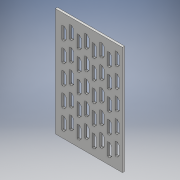
# Autodesk Inventor part: laminarFlowVOLUME50x31cm
Saved by Autodesk Inventor 2017 (Build 210142000, 142)
## iProperties
Created: 2018-08-04
Part Number: laminarFlowVOLUME50x31cm
Material: Generic
Document SubType Name: Modeling
Designer: qwertyuiop1
Density: 1 g/cm^3
Appearance: Default
Author: qwertyuiop1
Autodesk Inventor part; units mm, degrees
ref_plane "YZ Plane" through (0, 0, 0) normal (1, 0, 0) x (0, 1, 0)
ref_plane "XZ Plane" through (0, 0, 0) normal (0, 1, 0) x (-1, 0, 0)
ref_plane "XY Plane" through (0, 0, 0) normal (0, 0, 1) x (1, 0, 0)
sketch "Sketch1" plane through (0, 0, 0) normal (0, 1, 0) x (-1, 0, 0)
  line L0 (-32, 30) -> (-39.1716, 30)
  line L1 (-50, 40.8284) -> (-50, 79.1716)
  line L2 (-39.1716, 90) -> (-32, 90)
  line L3 (-30, 88) -> (-30, 32)
  line L4 (-49.4142, 80.5858) -> (-40.5858, 89.4142)
  line L5 (-40.5858, 30.5858) -> (-49.4142, 39.4142)
  arc A0 (-30, 88) -> (-32, 90) centre (-32, 88) ccw
  arc A1 (-39.1716, 90) -> (-40.5858, 89.4142) centre (-39.1716, 88) ccw
  arc A2 (-49.4142, 80.5858) -> (-50, 79.1716) centre (-48, 79.1716) ccw
  arc A3 (-50, 40.8284) -> (-49.4142, 39.4142) centre (-48, 40.8284) ccw
  arc A4 (-40.5858, 30.5858) -> (-39.1716, 30) centre (-39.1716, 32) ccw
  arc A5 (-32, 30) -> (-30, 32) centre (-32, 32) ccw
  line L6 (-32, 120) -> (-39.1716, 120)
  line L7 (-50, 130.8284) -> (-50, 169.1716)
  line L8 (-39.1716, 180) -> (-32, 180)
  line L9 (-30, 178) -> (-30, 122)
  line L10 (-49.4142, 170.5858) -> (-40.5858, 179.4142)
  line L11 (-40.5858, 120.5858) -> (-49.4142, 129.4142)
  arc A6 (-30, 178) -> (-32, 180) centre (-32, 178) ccw
  arc A7 (-39.1716, 180) -> (-40.5858, 179.4142) centre (-39.1716, 178) ccw
  arc A8 (-49.4142, 170.5858) -> (-50, 169.1716) centre (-48, 169.1716) ccw
  arc A9 (-50, 130.8284) -> (-49.4142, 129.4142) centre (-48, 130.8284) ccw
  arc A10 (-40.5858, 120.5858) -> (-39.1716, 120) centre (-39.1716, 122) ccw
  arc A11 (-32, 120) -> (-30, 122) centre (-32, 122) ccw
  line L12 (-32, 210) -> (-39.1716, 210)
  line L13 (-50, 220.8284) -> (-50, 259.1716)
  line L14 (-39.1716, 270) -> (-32, 270)
  line L15 (-30, 268) -> (-30, 212)
  line L16 (-49.4142, 260.5858) -> (-40.5858, 269.4142)
  line L17 (-40.5858, 210.5858) -> (-49.4142, 219.4142)
  arc A12 (-30, 268) -> (-32, 270) centre (-32, 268) ccw
  arc A13 (-39.1716, 270) -> (-40.5858, 269.4142) centre (-39.1716, 268) ccw
  arc A14 (-49.4142, 260.5858) -> (-50, 259.1716) centre (-48, 259.1716) ccw
  arc A15 (-50, 220.8284) -> (-49.4142, 219.4142) centre (-48, 220.8284) ccw
  arc A16 (-40.5858, 210.5858) -> (-39.1716, 210) centre (-39.1716, 212) ccw
  arc A17 (-32, 210) -> (-30, 212) centre (-32, 212) ccw
  line L18 (-32, 300) -> (-39.1716, 300)
  arc A18 (-50, 310.8284) -> (-49.4142, 309.4142) centre (-48, 310.8284) ccw
  arc A19 (-32, 300) -> (-30, 302) centre (-32, 302) ccw
  arc A20 (-40.5858, 300.5858) -> (-39.1716, 300) centre (-39.1716, 302) ccw
  line L19 (-40.5858, 300.5858) -> (-49.4142, 309.4142)
  line L20 (-50, 310.8284) -> (-50, 349.1716)
  line L21 (-30, 358) -> (-30, 302)
  arc A21 (-49.4142, 350.5858) -> (-50, 349.1716) centre (-48, 349.1716) ccw
  line L22 (-49.4142, 350.5858) -> (-40.5858, 359.4142)
  arc A22 (-39.1716, 360) -> (-40.5858, 359.4142) centre (-39.1716, 358) ccw
  line L23 (-39.1716, 360) -> (-32, 360)
  arc A23 (-30, 358) -> (-32, 360) centre (-32, 358) ccw
  line L24 (-32, 390) -> (-39.1716, 390)
  arc A24 (-40.5858, 390.5858) -> (-39.1716, 390) centre (-39.1716, 392) ccw
  arc A25 (-32, 390) -> (-30, 392) centre (-32, 392) ccw
  line L25 (-40.5858, 390.5858) -> (-49.4142, 399.4142)
  arc A26 (-50, 400.8284) -> (-49.4142, 399.4142) centre (-48, 400.8284) ccw
  line L26 (-30, 448) -> (-30, 392)
  line L27 (-50, 400.8284) -> (-50, 439.1716)
  arc A27 (-49.4142, 440.5858) -> (-50, 439.1716) centre (-48, 439.1716) ccw
  arc A28 (-30, 448) -> (-32, 450) centre (-32, 448) ccw
  line L28 (-39.1716, 450) -> (-32, 450)
  line L29 (-49.4142, 440.5858) -> (-40.5858, 449.4142)
  arc A29 (-39.1716, 450) -> (-40.5858, 449.4142) centre (-39.1716, 448) ccw
  line L30 (0, 0) -> (-309.0433, 0)
  line L31 (-309.0433, 0) -> (-309.0433, 500)
  line L32 (-309.0433, 500) -> (0, 500)
  line L33 (0, 500) -> (0, 0)
  line L34 (-67, 50) -> (-74.1716, 50)
  line L35 (-85, 60.8284) -> (-85, 99.1716)
  line L36 (-74.1716, 110) -> (-67, 110)
  line L37 (-65, 108) -> (-65, 52)
  line L38 (-84.4142, 100.5858) -> (-75.5858, 109.4142)
  line L39 (-75.5858, 50.5858) -> (-84.4142, 59.4142)
  arc A30 (-65, 108) -> (-67, 110) centre (-67, 108) ccw
  arc A31 (-74.1716, 110) -> (-75.5858, 109.4142) centre (-74.1716, 108) ccw
  arc A32 (-84.4142, 100.5858) -> (-85, 99.1716) centre (-83, 99.1716) ccw
  arc A33 (-85, 60.8284) -> (-84.4142, 59.4142) centre (-83, 60.8284) ccw
  arc A34 (-75.5858, 50.5858) -> (-74.1716, 50) centre (-74.1716, 52) ccw
  arc A35 (-67, 50) -> (-65, 52) centre (-67, 52) ccw
  line L40 (-67, 140) -> (-74.1716, 140)
  arc A36 (-85, 150.8284) -> (-84.4142, 149.4142) centre (-83, 150.8284) ccw
  arc A37 (-67, 140) -> (-65, 142) centre (-67, 142) ccw
  arc A38 (-75.5858, 140.5858) -> (-74.1716, 140) centre (-74.1716, 142) ccw
  line L41 (-75.5858, 140.5858) -> (-84.4142, 149.4142)
  line L42 (-85, 150.8284) -> (-85, 189.1716)
  line L43 (-65, 198) -> (-65, 142)
  arc A39 (-84.4142, 190.5858) -> (-85, 189.1716) centre (-83, 189.1716) ccw
  line L44 (-84.4142, 190.5858) -> (-75.5858, 199.4142)
  arc A40 (-74.1716, 200) -> (-75.5858, 199.4142) centre (-74.1716, 198) ccw
  line L45 (-74.1716, 200) -> (-67, 200)
  arc A41 (-65, 198) -> (-67, 200) centre (-67, 198) ccw
  line L46 (-67, 230) -> (-74.1716, 230)
  arc A42 (-85, 240.8284) -> (-84.4142, 239.4142) centre (-83, 240.8284) ccw
  arc A43 (-67, 230) -> (-65, 232) centre (-67, 232) ccw
  arc A44 (-75.5858, 230.5858) -> (-74.1716, 230) centre (-74.1716, 232) ccw
  line L47 (-75.5858, 230.5858) -> (-84.4142, 239.4142)
  line L48 (-85, 240.8284) -> (-85, 279.1716)
  line L49 (-65, 288) -> (-65, 232)
  arc A45 (-84.4142, 280.5858) -> (-85, 279.1716) centre (-83, 279.1716) ccw
  line L50 (-84.4142, 280.5858) -> (-75.5858, 289.4142)
  arc A46 (-74.1716, 290) -> (-75.5858, 289.4142) centre (-74.1716, 288) ccw
  line L51 (-74.1716, 290) -> (-67, 290)
  arc A47 (-65, 288) -> (-67, 290) centre (-67, 288) ccw
  line L52 (-67, 320) -> (-74.1716, 320)
  arc A48 (-75.5858, 320.5858) -> (-74.1716, 320) centre (-74.1716, 322) ccw
  arc A49 (-67, 320) -> (-65, 322) centre (-67, 322) ccw
  line L53 (-75.5858, 320.5858) -> (-84.4142, 329.4142)
  arc A50 (-85, 330.8284) -> (-84.4142, 329.4142) centre (-83, 330.8284) ccw
  line L54 (-65, 378) -> (-65, 322)
  line L55 (-85, 330.8284) -> (-85, 369.1716)
  arc A51 (-84.4142, 370.5858) -> (-85, 369.1716) centre (-83, 369.1716) ccw
  arc A52 (-65, 378) -> (-67, 380) centre (-67, 378) ccw
  line L56 (-74.1716, 380) -> (-67, 380)
  line L57 (-84.4142, 370.5858) -> (-75.5858, 379.4142)
  arc A53 (-74.1716, 380) -> (-75.5858, 379.4142) centre (-74.1716, 378) ccw
  line L58 (-67, 410) -> (-74.1716, 410)
  arc A54 (-75.5858, 410.5858) -> (-74.1716, 410) centre (-74.1716, 412) ccw
  arc A55 (-67, 410) -> (-65, 412) centre (-67, 412) ccw
  line L59 (-75.5858, 410.5858) -> (-84.4142, 419.4142)
  line L60 (-65, 468) -> (-65, 412)
  line L61 (-85, 420.8284) -> (-85, 459.1716)
  arc A56 (-85, 420.8284) -> (-84.4142, 419.4142) centre (-83, 420.8284) ccw
  arc A57 (-84.4142, 460.5858) -> (-85, 459.1716) centre (-83, 459.1716) ccw
  line L62 (-84.4142, 460.5858) -> (-75.5858, 469.4142)
  arc A58 (-74.1716, 470) -> (-75.5858, 469.4142) centre (-74.1716, 468) ccw
  line L63 (-74.1716, 470) -> (-67, 470)
  arc A59 (-65, 468) -> (-67, 470) centre (-67, 468) ccw
  line L64 (-102, 30) -> (-109.1716, 30)
  line L65 (-120, 40.8284) -> (-120, 79.1716)
  line L66 (-109.1716, 90) -> (-102, 90)
  line L67 (-100, 88) -> (-100, 32)
  line L68 (-119.4142, 80.5858) -> (-110.5858, 89.4142)
  line L69 (-110.5858, 30.5858) -> (-119.4142, 39.4142)
  arc A60 (-100, 88) -> (-102, 90) centre (-102, 88) ccw
  arc A61 (-109.1716, 90) -> (-110.5858, 89.4142) centre (-109.1716, 88) ccw
  arc A62 (-119.4142, 80.5858) -> (-120, 79.1716) centre (-118, 79.1716) ccw
  arc A63 (-120, 40.8284) -> (-119.4142, 39.4142) centre (-118, 40.8284) ccw
  arc A64 (-110.5858, 30.5858) -> (-109.1716, 30) centre (-109.1716, 32) ccw
  arc A65 (-102, 30) -> (-100, 32) centre (-102, 32) ccw
  line L70 (-102, 120) -> (-109.1716, 120)
  arc A66 (-120, 130.8284) -> (-119.4142, 129.4142) centre (-118, 130.8284) ccw
  arc A67 (-102, 120) -> (-100, 122) centre (-102, 122) ccw
  arc A68 (-110.5858, 120.5858) -> (-109.1716, 120) centre (-109.1716, 122) ccw
  line L71 (-110.5858, 120.5858) -> (-119.4142, 129.4142)
  line L72 (-120, 130.8284) -> (-120, 169.1716)
  line L73 (-100, 178) -> (-100, 122)
  arc A69 (-119.4142, 170.5858) -> (-120, 169.1716) centre (-118, 169.1716) ccw
  line L74 (-119.4142, 170.5858) -> (-110.5858, 179.4142)
  arc A70 (-109.1716, 180) -> (-110.5858, 179.4142) centre (-109.1716, 178) ccw
  line L75 (-109.1716, 180) -> (-102, 180)
  arc A71 (-100, 178) -> (-102, 180) centre (-102, 178) ccw
  line L76 (-102, 210) -> (-109.1716, 210)
  arc A72 (-120, 220.8284) -> (-119.4142, 219.4142) centre (-118, 220.8284) ccw
  arc A73 (-102, 210) -> (-100, 212) centre (-102, 212) ccw
  arc A74 (-110.5858, 210.5858) -> (-109.1716, 210) centre (-109.1716, 212) ccw
  line L77 (-110.5858, 210.5858) -> (-119.4142, 219.4142)
  line L78 (-120, 220.8284) -> (-120, 259.1716)
  line L79 (-100, 268) -> (-100, 212)
  arc A75 (-119.4142, 260.5858) -> (-120, 259.1716) centre (-118, 259.1716) ccw
  line L80 (-119.4142, 260.5858) -> (-110.5858, 269.4142)
  arc A76 (-109.1716, 270) -> (-110.5858, 269.4142) centre (-109.1716, 268) ccw
  line L81 (-109.1716, 270) -> (-102, 270)
  arc A77 (-100, 268) -> (-102, 270) centre (-102, 268) ccw
  line L82 (-102, 300) -> (-109.1716, 300)
  arc A78 (-110.5858, 300.5858) -> (-109.1716, 300) centre (-109.1716, 302) ccw
  arc A79 (-102, 300) -> (-100, 302) centre (-102, 302) ccw
  line L83 (-110.5858, 300.5858) -> (-119.4142, 309.4142)
  arc A80 (-120, 310.8284) -> (-119.4142, 309.4142) centre (-118, 310.8284) ccw
  line L84 (-100, 358) -> (-100, 302)
  line L85 (-120, 310.8284) -> (-120, 349.1716)
  arc A81 (-119.4142, 350.5858) -> (-120, 349.1716) centre (-118, 349.1716) ccw
  arc A82 (-100, 358) -> (-102, 360) centre (-102, 358) ccw
  line L86 (-109.1716, 360) -> (-102, 360)
  line L87 (-119.4142, 350.5858) -> (-110.5858, 359.4142)
  arc A83 (-109.1716, 360) -> (-110.5858, 359.4142) centre (-109.1716, 358) ccw
  line L88 (-102, 390) -> (-109.1716, 390)
  arc A84 (-110.5858, 390.5858) -> (-109.1716, 390) centre (-109.1716, 392) ccw
  arc A85 (-102, 390) -> (-100, 392) centre (-102, 392) ccw
  line L89 (-110.5858, 390.5858) -> (-119.4142, 399.4142)
  line L90 (-100, 448) -> (-100, 392)
  line L91 (-120, 400.8284) -> (-120, 439.1716)
  arc A86 (-120, 400.8284) -> (-119.4142, 399.4142) centre (-118, 400.8284) ccw
  arc A87 (-119.4142, 440.5858) -> (-120, 439.1716) centre (-118, 439.1716) ccw
  line L92 (-119.4142, 440.5858) -> (-110.5858, 449.4142)
  arc A88 (-109.1716, 450) -> (-110.5858, 449.4142) centre (-109.1716, 448) ccw
  line L93 (-109.1716, 450) -> (-102, 450)
  arc A89 (-100, 448) -> (-102, 450) centre (-102, 448) ccw
  arc A90 (-155, 420.8284) -> (-154.4142, 419.4142) centre (-153, 420.8284) ccw
  line L94 (-155, 420.8284) -> (-155, 459.1716)
  line L95 (-135, 468) -> (-135, 412)
  line L96 (-144.1716, 470) -> (-137, 470)
  arc A91 (-145.5858, 410.5858) -> (-144.1716, 410) centre (-144.1716, 412) ccw
  arc A92 (-137, 410) -> (-135, 412) centre (-137, 412) ccw
  line L97 (-145.5858, 410.5858) -> (-154.4142, 419.4142)
  arc A93 (-154.4142, 460.5858) -> (-155, 459.1716) centre (-153, 459.1716) ccw
  line L98 (-154.4142, 460.5858) -> (-145.5858, 469.4142)
  arc A94 (-135, 468) -> (-137, 470) centre (-137, 468) ccw
  arc A95 (-144.1716, 470) -> (-145.5858, 469.4142) centre (-144.1716, 468) ccw
  line L99 (-137, 50) -> (-144.1716, 50)
  arc A96 (-154.4142, 280.5858) -> (-155, 279.1716) centre (-153, 279.1716) ccw
  line L100 (-154.4142, 280.5858) -> (-145.5858, 289.4142)
  arc A97 (-144.1716, 290) -> (-145.5858, 289.4142) centre (-144.1716, 288) ccw
  arc A98 (-154.4142, 370.5858) -> (-155, 369.1716) centre (-153, 369.1716) ccw
  arc A99 (-155, 330.8284) -> (-154.4142, 329.4142) centre (-153, 330.8284) ccw
  arc A100 (-144.1716, 380) -> (-145.5858, 379.4142) centre (-144.1716, 378) ccw
  line L101 (-145.5858, 50.5858) -> (-154.4142, 59.4142)
  line L102 (-155, 60.8284) -> (-155, 99.1716)
  line L103 (-154.4142, 100.5858) -> (-145.5858, 109.4142)
  line L104 (-135, 108) -> (-135, 52)
  line L105 (-144.1716, 110) -> (-137, 110)
  line L106 (-155, 330.8284) -> (-155, 369.1716)
  line L107 (-144.1716, 290) -> (-137, 290)
  line L108 (-137, 320) -> (-144.1716, 320)
  line L109 (-137, 410) -> (-144.1716, 410)
  arc A101 (-137, 320) -> (-135, 322) centre (-137, 322) ccw
  arc A102 (-135, 288) -> (-137, 290) centre (-137, 288) ccw
  line L110 (-154.4142, 370.5858) -> (-145.5858, 379.4142)
  line L111 (-145.5858, 320.5858) -> (-154.4142, 329.4142)
  arc A103 (-135, 378) -> (-137, 380) centre (-137, 378) ccw
  arc A104 (-135, 108) -> (-137, 110) centre (-137, 108) ccw
  arc A105 (-144.1716, 110) -> (-145.5858, 109.4142) centre (-144.1716, 108) ccw
  arc A106 (-154.4142, 100.5858) -> (-155, 99.1716) centre (-153, 99.1716) ccw
  arc A107 (-155, 240.8284) -> (-154.4142, 239.4142) centre (-153, 240.8284) ccw
  arc A108 (-155, 60.8284) -> (-154.4142, 59.4142) centre (-153, 60.8284) ccw
  arc A109 (-145.5858, 50.5858) -> (-144.1716, 50) centre (-144.1716, 52) ccw
  arc A110 (-137, 50) -> (-135, 52) centre (-137, 52) ccw
  line L112 (-135, 378) -> (-135, 322)
  line L113 (-144.1716, 380) -> (-137, 380)
  line L114 (-137, 230) -> (-144.1716, 230)
  line L115 (-155, 240.8284) -> (-155, 279.1716)
  line L116 (-145.5858, 230.5858) -> (-154.4142, 239.4142)
  line L117 (-135, 288) -> (-135, 232)
  line L118 (-155, 150.8284) -> (-155, 189.1716)
  line L119 (-135, 198) -> (-135, 142)
  line L120 (-145.5858, 140.5858) -> (-154.4142, 149.4142)
  arc A111 (-155, 150.8284) -> (-154.4142, 149.4142) centre (-153, 150.8284) ccw
  arc A112 (-137, 140) -> (-135, 142) centre (-137, 142) ccw
  arc A113 (-145.5858, 140.5858) -> (-144.1716, 140) centre (-144.1716, 142) ccw
  line L121 (-137, 140) -> (-144.1716, 140)
  arc A114 (-145.5858, 320.5858) -> (-144.1716, 320) centre (-144.1716, 322) ccw
  arc A115 (-137, 230) -> (-135, 232) centre (-137, 232) ccw
  arc A116 (-145.5858, 230.5858) -> (-144.1716, 230) centre (-144.1716, 232) ccw
  line L122 (-144.1716, 200) -> (-137, 200)
  arc A117 (-144.1716, 200) -> (-145.5858, 199.4142) centre (-144.1716, 198) ccw
  arc A118 (-135, 198) -> (-137, 200) centre (-137, 198) ccw
  line L123 (-154.4142, 190.5858) -> (-145.5858, 199.4142)
  arc A119 (-154.4142, 190.5858) -> (-155, 189.1716) centre (-153, 189.1716) ccw
  line L124 (-172, 30) -> (-179.1716, 30)
  line L125 (-190, 40.8284) -> (-190, 79.1716)
  line L126 (-179.1716, 90) -> (-172, 90)
  line L127 (-170, 88) -> (-170, 32)
  line L128 (-189.4142, 80.5858) -> (-180.5858, 89.4142)
  line L129 (-180.5858, 30.5858) -> (-189.4142, 39.4142)
  arc A120 (-170, 88) -> (-172, 90) centre (-172, 88) ccw
  arc A121 (-179.1716, 90) -> (-180.5858, 89.4142) centre (-179.1716, 88) ccw
  arc A122 (-189.4142, 80.5858) -> (-190, 79.1716) centre (-188, 79.1716) ccw
  arc A123 (-190, 40.8284) -> (-189.4142, 39.4142) centre (-188, 40.8284) ccw
  arc A124 (-180.5858, 30.5858) -> (-179.1716, 30) centre (-179.1716, 32) ccw
  arc A125 (-172, 30) -> (-170, 32) centre (-172, 32) ccw
  line L130 (-172, 120) -> (-179.1716, 120)
  arc A126 (-190, 130.8284) -> (-189.4142, 129.4142) centre (-188, 130.8284) ccw
  arc A127 (-172, 120) -> (-170, 122) centre (-172, 122) ccw
  arc A128 (-180.5858, 120.5858) -> (-179.1716, 120) centre (-179.1716, 122) ccw
  line L131 (-180.5858, 120.5858) -> (-189.4142, 129.4142)
  line L132 (-190, 130.8284) -> (-190, 169.1716)
  line L133 (-170, 178) -> (-170, 122)
  arc A129 (-189.4142, 170.5858) -> (-190, 169.1716) centre (-188, 169.1716) ccw
  line L134 (-189.4142, 170.5858) -> (-180.5858, 179.4142)
  arc A130 (-179.1716, 180) -> (-180.5858, 179.4142) centre (-179.1716, 178) ccw
  line L135 (-179.1716, 180) -> (-172, 180)
  arc A131 (-170, 178) -> (-172, 180) centre (-172, 178) ccw
  line L136 (-172, 210) -> (-179.1716, 210)
  arc A132 (-190, 220.8284) -> (-189.4142, 219.4142) centre (-188, 220.8284) ccw
  arc A133 (-172, 210) -> (-170, 212) centre (-172, 212) ccw
  arc A134 (-180.5858, 210.5858) -> (-179.1716, 210) centre (-179.1716, 212) ccw
  line L137 (-180.5858, 210.5858) -> (-189.4142, 219.4142)
  line L138 (-190, 220.8284) -> (-190, 259.1716)
  line L139 (-170, 268) -> (-170, 212)
  arc A135 (-189.4142, 260.5858) -> (-190, 259.1716) centre (-188, 259.1716) ccw
  line L140 (-189.4142, 260.5858) -> (-180.5858, 269.4142)
  arc A136 (-179.1716, 270) -> (-180.5858, 269.4142) centre (-179.1716, 268) ccw
  line L141 (-179.1716, 270) -> (-172, 270)
  arc A137 (-170, 268) -> (-172, 270) centre (-172, 268) ccw
  line L142 (-172, 300) -> (-179.1716, 300)
  arc A138 (-180.5858, 300.5858) -> (-179.1716, 300) centre (-179.1716, 302) ccw
  arc A139 (-172, 300) -> (-170, 302) centre (-172, 302) ccw
  line L143 (-180.5858, 300.5858) -> (-189.4142, 309.4142)
  arc A140 (-190, 310.8284) -> (-189.4142, 309.4142) centre (-188, 310.8284) ccw
  line L144 (-170, 358) -> (-170, 302)
  line L145 (-190, 310.8284) -> (-190, 349.1716)
  arc A141 (-189.4142, 350.5858) -> (-190, 349.1716) centre (-188, 349.1716) ccw
  arc A142 (-170, 358) -> (-172, 360) centre (-172, 358) ccw
  line L146 (-179.1716, 360) -> (-172, 360)
  line L147 (-189.4142, 350.5858) -> (-180.5858, 359.4142)
  arc A143 (-179.1716, 360) -> (-180.5858, 359.4142) centre (-179.1716, 358) ccw
  line L148 (-172, 390) -> (-179.1716, 390)
  arc A144 (-180.5858, 390.5858) -> (-179.1716, 390) centre (-179.1716, 392) ccw
  arc A145 (-172, 390) -> (-170, 392) centre (-172, 392) ccw
  line L149 (-180.5858, 390.5858) -> (-189.4142, 399.4142)
  line L150 (-170, 448) -> (-170, 392)
  line L151 (-190, 400.8284) -> (-190, 439.1716)
  arc A146 (-190, 400.8284) -> (-189.4142, 399.4142) centre (-188, 400.8284) ccw
  arc A147 (-189.4142, 440.5858) -> (-190, 439.1716) centre (-188, 439.1716) ccw
  line L152 (-189.4142, 440.5858) -> (-180.5858, 449.4142)
  arc A148 (-179.1716, 450) -> (-180.5858, 449.4142) centre (-179.1716, 448) ccw
  line L153 (-179.1716, 450) -> (-172, 450)
  arc A149 (-170, 448) -> (-172, 450) centre (-172, 448) ccw
  arc A150 (-225, 420.8284) -> (-224.4142, 419.4142) centre (-223, 420.8284) ccw
  line L154 (-225, 420.8284) -> (-225, 459.1716)
  line L155 (-205, 468) -> (-205, 412)
  line L156 (-214.1716, 470) -> (-207, 470)
  arc A151 (-215.5858, 410.5858) -> (-214.1716, 410) centre (-214.1716, 412) ccw
  arc A152 (-207, 410) -> (-205, 412) centre (-207, 412) ccw
  line L157 (-215.5858, 410.5858) -> (-224.4142, 419.4142)
  arc A153 (-224.4142, 460.5858) -> (-225, 459.1716) centre (-223, 459.1716) ccw
  line L158 (-224.4142, 460.5858) -> (-215.5858, 469.4142)
  arc A154 (-205, 468) -> (-207, 470) centre (-207, 468) ccw
  arc A155 (-214.1716, 470) -> (-215.5858, 469.4142) centre (-214.1716, 468) ccw
  line L159 (-207, 50) -> (-214.1716, 50)
  arc A156 (-224.4142, 280.5858) -> (-225, 279.1716) centre (-223, 279.1716) ccw
  line L160 (-224.4142, 280.5858) -> (-215.5858, 289.4142)
  arc A157 (-214.1716, 290) -> (-215.5858, 289.4142) centre (-214.1716, 288) ccw
  arc A158 (-224.4142, 370.5858) -> (-225, 369.1716) centre (-223, 369.1716) ccw
  arc A159 (-225, 330.8284) -> (-224.4142, 329.4142) centre (-223, 330.8284) ccw
  arc A160 (-214.1716, 380) -> (-215.5858, 379.4142) centre (-214.1716, 378) ccw
  line L161 (-215.5858, 50.5858) -> (-224.4142, 59.4142)
  line L162 (-225, 60.8284) -> (-225, 99.1716)
  line L163 (-224.4142, 100.5858) -> (-215.5858, 109.4142)
  line L164 (-205, 108) -> (-205, 52)
  line L165 (-214.1716, 110) -> (-207, 110)
  line L166 (-225, 330.8284) -> (-225, 369.1716)
  line L167 (-214.1716, 290) -> (-207, 290)
  line L168 (-207, 320) -> (-214.1716, 320)
  line L169 (-207, 410) -> (-214.1716, 410)
  arc A161 (-207, 320) -> (-205, 322) centre (-207, 322) ccw
  arc A162 (-205, 288) -> (-207, 290) centre (-207, 288) ccw
  line L170 (-224.4142, 370.5858) -> (-215.5858, 379.4142)
  line L171 (-215.5858, 320.5858) -> (-224.4142, 329.4142)
  arc A163 (-205, 378) -> (-207, 380) centre (-207, 378) ccw
  arc A164 (-205, 108) -> (-207, 110) centre (-207, 108) ccw
  arc A165 (-214.1716, 110) -> (-215.5858, 109.4142) centre (-214.1716, 108) ccw
  arc A166 (-224.4142, 100.5858) -> (-225, 99.1716) centre (-223, 99.1716) ccw
  arc A167 (-225, 240.8284) -> (-224.4142, 239.4142) centre (-223, 240.8284) ccw
  arc A168 (-225, 60.8284) -> (-224.4142, 59.4142) centre (-223, 60.8284) ccw
  arc A169 (-215.5858, 50.5858) -> (-214.1716, 50) centre (-214.1716, 52) ccw
  arc A170 (-207, 50) -> (-205, 52) centre (-207, 52) ccw
  line L172 (-205, 378) -> (-205, 322)
  line L173 (-214.1716, 380) -> (-207, 380)
  line L174 (-207, 230) -> (-214.1716, 230)
  line L175 (-225, 240.8284) -> (-225, 279.1716)
  line L176 (-215.5858, 230.5858) -> (-224.4142, 239.4142)
  line L177 (-205, 288) -> (-205, 232)
  line L178 (-225, 150.8284) -> (-225, 189.1716)
  line L179 (-205, 198) -> (-205, 142)
  line L180 (-215.5858, 140.5858) -> (-224.4142, 149.4142)
  arc A171 (-225, 150.8284) -> (-224.4142, 149.4142) centre (-223, 150.8284) ccw
  arc A172 (-207, 140) -> (-205, 142) centre (-207, 142) ccw
  arc A173 (-215.5858, 140.5858) -> (-214.1716, 140) centre (-214.1716, 142) ccw
  line L181 (-207, 140) -> (-214.1716, 140)
  arc A174 (-215.5858, 320.5858) -> (-214.1716, 320) centre (-214.1716, 322) ccw
  arc A175 (-207, 230) -> (-205, 232) centre (-207, 232) ccw
  arc A176 (-215.5858, 230.5858) -> (-214.1716, 230) centre (-214.1716, 232) ccw
  line L182 (-214.1716, 200) -> (-207, 200)
  arc A177 (-214.1716, 200) -> (-215.5858, 199.4142) centre (-214.1716, 198) ccw
  arc A178 (-205, 198) -> (-207, 200) centre (-207, 198) ccw
  line L183 (-224.4142, 190.5858) -> (-215.5858, 199.4142)
  arc A179 (-224.4142, 190.5858) -> (-225, 189.1716) centre (-223, 189.1716) ccw
  line L184 (-242, 30) -> (-249.1716, 30)
  line L185 (-260, 40.8284) -> (-260, 79.1716)
  line L186 (-249.1716, 90) -> (-242, 90)
  line L187 (-240, 88) -> (-240, 32)
  line L188 (-259.4142, 80.5858) -> (-250.5858, 89.4142)
  line L189 (-250.5858, 30.5858) -> (-259.4142, 39.4142)
  arc A180 (-240, 88) -> (-242, 90) centre (-242, 88) ccw
  arc A181 (-249.1716, 90) -> (-250.5858, 89.4142) centre (-249.1716, 88) ccw
  arc A182 (-259.4142, 80.5858) -> (-260, 79.1716) centre (-258, 79.1716) ccw
  arc A183 (-260, 40.8284) -> (-259.4142, 39.4142) centre (-258, 40.8284) ccw
  arc A184 (-250.5858, 30.5858) -> (-249.1716, 30) centre (-249.1716, 32) ccw
  arc A185 (-242, 30) -> (-240, 32) centre (-242, 32) ccw
  line L190 (-242, 120) -> (-249.1716, 120)
  arc A186 (-260, 130.8284) -> (-259.4142, 129.4142) centre (-258, 130.8284) ccw
  arc A187 (-242, 120) -> (-240, 122) centre (-242, 122) ccw
  arc A188 (-250.5858, 120.5858) -> (-249.1716, 120) centre (-249.1716, 122) ccw
  line L191 (-250.5858, 120.5858) -> (-259.4142, 129.4142)
  line L192 (-260, 130.8284) -> (-260, 169.1716)
  line L193 (-240, 178) -> (-240, 122)
  arc A189 (-259.4142, 170.5858) -> (-260, 169.1716) centre (-258, 169.1716) ccw
  line L194 (-259.4142, 170.5858) -> (-250.5858, 179.4142)
  arc A190 (-249.1716, 180) -> (-250.5858, 179.4142) centre (-249.1716, 178) ccw
  line L195 (-249.1716, 180) -> (-242, 180)
  arc A191 (-240, 178) -> (-242, 180) centre (-242, 178) ccw
  line L196 (-242, 210) -> (-249.1716, 210)
  arc A192 (-260, 220.8284) -> (-259.4142, 219.4142) centre (-258, 220.8284) ccw
  arc A193 (-242, 210) -> (-240, 212) centre (-242, 212) ccw
  arc A194 (-250.5858, 210.5858) -> (-249.1716, 210) centre (-249.1716, 212) ccw
  line L197 (-250.5858, 210.5858) -> (-259.4142, 219.4142)
  line L198 (-260, 220.8284) -> (-260, 259.1716)
  line L199 (-240, 268) -> (-240, 212)
  arc A195 (-259.4142, 260.5858) -> (-260, 259.1716) centre (-258, 259.1716) ccw
  line L200 (-259.4142, 260.5858) -> (-250.5858, 269.4142)
  arc A196 (-249.1716, 270) -> (-250.5858, 269.4142) centre (-249.1716, 268) ccw
  line L201 (-249.1716, 270) -> (-242, 270)
  arc A197 (-240, 268) -> (-242, 270) centre (-242, 268) ccw
  line L202 (-242, 300) -> (-249.1716, 300)
  arc A198 (-250.5858, 300.5858) -> (-249.1716, 300) centre (-249.1716, 302) ccw
  arc A199 (-242, 300) -> (-240, 302) centre (-242, 302) ccw
  line L203 (-250.5858, 300.5858) -> (-259.4142, 309.4142)
  arc A200 (-260, 310.8284) -> (-259.4142, 309.4142) centre (-258, 310.8284) ccw
  line L204 (-240, 358) -> (-240, 302)
  line L205 (-260, 310.8284) -> (-260, 349.1716)
  arc A201 (-259.4142, 350.5858) -> (-260, 349.1716) centre (-258, 349.1716) ccw
  arc A202 (-240, 358) -> (-242, 360) centre (-242, 358) ccw
  line L206 (-249.1716, 360) -> (-242, 360)
  line L207 (-259.4142, 350.5858) -> (-250.5858, 359.4142)
  arc A203 (-249.1716, 360) -> (-250.5858, 359.4142) centre (-249.1716, 358) ccw
  line L208 (-242, 390) -> (-249.1716, 390)
  arc A204 (-250.5858, 390.5858) -> (-249.1716, 390) centre (-249.1716, 392) ccw
  arc A205 (-242, 390) -> (-240, 392) centre (-242, 392) ccw
  line L209 (-250.5858, 390.5858) -> (-259.4142, 399.4142)
  line L210 (-240, 448) -> (-240, 392)
  line L211 (-260, 400.8284) -> (-260, 439.1716)
  arc A206 (-260, 400.8284) -> (-259.4142, 399.4142) centre (-258, 400.8284) ccw
  arc A207 (-259.4142, 440.5858) -> (-260, 439.1716) centre (-258, 439.1716) ccw
  line L212 (-259.4142, 440.5858) -> (-250.5858, 449.4142)
  arc A208 (-249.1716, 450) -> (-250.5858, 449.4142) centre (-249.1716, 448) ccw
  line L213 (-249.1716, 450) -> (-242, 450)
  arc A209 (-240, 448) -> (-242, 450) centre (-242, 448) ccw
  arc A210 (-295, 420.8284) -> (-294.4142, 419.4142) centre (-293, 420.8284) ccw
  line L214 (-295, 420.8284) -> (-295, 459.1716)
  line L215 (-275, 468) -> (-275, 412)
  line L216 (-284.1716, 470) -> (-277, 470)
  arc A211 (-285.5858, 410.5858) -> (-284.1716, 410) centre (-284.1716, 412) ccw
  arc A212 (-277, 410) -> (-275, 412) centre (-277, 412) ccw
  line L217 (-285.5858, 410.5858) -> (-294.4142, 419.4142)
  arc A213 (-294.4142, 460.5858) -> (-295, 459.1716) centre (-293, 459.1716) ccw
  line L218 (-294.4142, 460.5858) -> (-285.5858, 469.4142)
  arc A214 (-275, 468) -> (-277, 470) centre (-277, 468) ccw
  arc A215 (-284.1716, 470) -> (-285.5858, 469.4142) centre (-284.1716, 468) ccw
  line L219 (-277, 50) -> (-284.1716, 50)
  arc A216 (-294.4142, 280.5858) -> (-295, 279.1716) centre (-293, 279.1716) ccw
  line L220 (-294.4142, 280.5858) -> (-285.5858, 289.4142)
  arc A217 (-284.1716, 290) -> (-285.5858, 289.4142) centre (-284.1716, 288) ccw
  arc A218 (-294.4142, 370.5858) -> (-295, 369.1716) centre (-293, 369.1716) ccw
  arc A219 (-295, 330.8284) -> (-294.4142, 329.4142) centre (-293, 330.8284) ccw
  arc A220 (-284.1716, 380) -> (-285.5858, 379.4142) centre (-284.1716, 378) ccw
  line L221 (-285.5858, 50.5858) -> (-294.4142, 59.4142)
  line L222 (-295, 60.8284) -> (-295, 99.1716)
  line L223 (-294.4142, 100.5858) -> (-285.5858, 109.4142)
  line L224 (-275, 108) -> (-275, 52)
  line L225 (-284.1716, 110) -> (-277, 110)
  line L226 (-295, 330.8284) -> (-295, 369.1716)
  line L227 (-284.1716, 290) -> (-277, 290)
  line L228 (-277, 320) -> (-284.1716, 320)
  line L229 (-277, 410) -> (-284.1716, 410)
  arc A221 (-277, 320) -> (-275, 322) centre (-277, 322) ccw
  arc A222 (-275, 288) -> (-277, 290) centre (-277, 288) ccw
  line L230 (-294.4142, 370.5858) -> (-285.5858, 379.4142)
  line L231 (-285.5858, 320.5858) -> (-294.4142, 329.4142)
  arc A223 (-275, 378) -> (-277, 380) centre (-277, 378) ccw
  arc A224 (-275, 108) -> (-277, 110) centre (-277, 108) ccw
  arc A225 (-284.1716, 110) -> (-285.5858, 109.4142) centre (-284.1716, 108) ccw
  arc A226 (-294.4142, 100.5858) -> (-295, 99.1716) centre (-293, 99.1716) ccw
  arc A227 (-295, 240.8284) -> (-294.4142, 239.4142) centre (-293, 240.8284) ccw
  arc A228 (-295, 60.8284) -> (-294.4142, 59.4142) centre (-293, 60.8284) ccw
  arc A229 (-285.5858, 50.5858) -> (-284.1716, 50) centre (-284.1716, 52) ccw
  arc A230 (-277, 50) -> (-275, 52) centre (-277, 52) ccw
  line L232 (-275, 378) -> (-275, 322)
  line L233 (-284.1716, 380) -> (-277, 380)
  line L234 (-277, 230) -> (-284.1716, 230)
  line L235 (-295, 240.8284) -> (-295, 279.1716)
  line L236 (-285.5858, 230.5858) -> (-294.4142, 239.4142)
  line L237 (-275, 288) -> (-275, 232)
  line L238 (-295, 150.8284) -> (-295, 189.1716)
  line L239 (-275, 198) -> (-275, 142)
  line L240 (-285.5858, 140.5858) -> (-294.4142, 149.4142)
  arc A231 (-295, 150.8284) -> (-294.4142, 149.4142) centre (-293, 150.8284) ccw
  arc A232 (-277, 140) -> (-275, 142) centre (-277, 142) ccw
  arc A233 (-285.5858, 140.5858) -> (-284.1716, 140) centre (-284.1716, 142) ccw
  line L241 (-277, 140) -> (-284.1716, 140)
  arc A234 (-285.5858, 320.5858) -> (-284.1716, 320) centre (-284.1716, 322) ccw
  arc A235 (-277, 230) -> (-275, 232) centre (-277, 232) ccw
  arc A236 (-285.5858, 230.5858) -> (-284.1716, 230) centre (-284.1716, 232) ccw
  line L242 (-284.1716, 200) -> (-277, 200)
  arc A237 (-284.1716, 200) -> (-285.5858, 199.4142) centre (-284.1716, 198) ccw
  arc A238 (-275, 198) -> (-277, 200) centre (-277, 198) ccw
  line L243 (-294.4142, 190.5858) -> (-285.5858, 199.4142)
  arc A239 (-294.4142, 190.5858) -> (-295, 189.1716) centre (-293, 189.1716) ccw
  point P0 (-50, 90)
  point P1 (-50, 30)
  point P2 (-30, 90)
  point P3 (-50, 80)
  point P4 (-40, 90)
  point P5 (-40, 30)
  point P6 (-50, 40)
  point P7 (-32, 180)
  point P8 (-32, 155.0655)
  point P9 (-32, 392)
  point P10 (-50, 180)
  point P11 (-50, 120)
  point P12 (-30, 180)
  point P13 (-50, 170)
  point P14 (-40, 180)
  point P15 (-40, 120)
  point P16 (-50, 130)
  point P17 (-50, 270)
  point P18 (-50, 210)
  point P19 (-30, 270)
  point P20 (-50, 260)
  point P21 (-40, 270)
  point P22 (-40, 210)
  point P23 (-50, 220)
  point P24 (-50, 300)
  point P25 (-50, 310)
  point P26 (-40, 300)
  point P27 (-50, 360)
  point P28 (-30, 360)
  point P29 (-50, 350)
  point P30 (-40, 360)
  point P31 (-40, 390)
  point P32 (-50, 390)
  point P33 (-50, 400)
  point P34 (-30, 450)
  point P35 (-40, 450)
  point P36 (-50, 450)
  point P37 (-50, 440)
  point P38 (-85, 50)
  point P39 (-85, 110)
  point P40 (-85, 50)
  point P41 (-65, 110)
  point P42 (-85, 100)
  point P43 (-75, 110)
  point P44 (-75, 50)
  point P45 (-85, 60)
  point P46 (-67, 200)
  point P47 (-67, 175.0655)
  point P48 (-67, 412)
  point P49 (-85, 140)
  point P50 (-85, 150)
  point P51 (-75, 140)
  point P52 (-85, 200)
  point P53 (-65, 200)
  point P54 (-85, 190)
  point P55 (-75, 200)
  point P56 (-85, 230)
  point P57 (-85, 240)
  point P58 (-75, 230)
  point P59 (-85, 290)
  point P60 (-65, 290)
  point P61 (-85, 280)
  point P62 (-75, 290)
  point P63 (-75, 320)
  point P64 (-85, 320)
  point P65 (-85, 330)
  point P66 (-65, 380)
  point P67 (-75, 380)
  point P68 (-85, 380)
  point P69 (-85, 370)
  point P70 (-75, 410)
  point P71 (-85, 410)
  point P72 (-85, 420)
  point P73 (-85, 460)
  point P74 (-85, 470)
  point P75 (-75, 470)
  point P76 (-65, 470)
  point P77 (-120, 30)
  point P78 (-120, 90)
  point P79 (-120, 30)
  point P80 (-100, 90)
  point P81 (-120, 80)
  point P82 (-110, 90)
  point P83 (-110, 30)
  point P84 (-120, 40)
  point P85 (-102, 180)
  point P86 (-102, 155.0655)
  point P87 (-102, 392)
  point P88 (-120, 120)
  point P89 (-120, 130)
  point P90 (-110, 120)
  point P91 (-120, 180)
  point P92 (-100, 180)
  point P93 (-120, 170)
  point P94 (-110, 180)
  point P95 (-120, 210)
  point P96 (-120, 220)
  point P97 (-110, 210)
  point P98 (-120, 270)
  point P99 (-100, 270)
  point P100 (-120, 260)
  point P101 (-110, 270)
  point P102 (-110, 300)
  point P103 (-120, 300)
  point P104 (-120, 310)
  point P105 (-100, 360)
  point P106 (-110, 360)
  point P107 (-120, 360)
  point P108 (-120, 350)
  point P109 (-110, 390)
  point P110 (-120, 390)
  point P111 (-120, 400)
  point P112 (-120, 440)
  point P113 (-120, 450)
  point P114 (-110, 450)
  point P115 (-100, 450)
  point P116 (-155, 50)
  point P117 (-155, 420)
  point P118 (-155, 470)
  point P119 (-135, 470)
  point P120 (-155, 460)
  point P121 (-145, 470)
  point P122 (-145, 50)
  point P123 (-155, 50)
  point P124 (-155, 290)
  point P125 (-145, 380)
  point P126 (-155, 380)
  point P127 (-155, 410)
  point P128 (-155, 370)
  point P129 (-155, 60)
  point P130 (-155, 100)
  point P131 (-145, 110)
  point P132 (-155, 110)
  point P133 (-135, 110)
  point P134 (-145, 320)
  point P135 (-155, 330)
  point P136 (-155, 320)
  point P137 (-145, 410)
  point P138 (-135, 290)
  point P139 (-145, 290)
  point P140 (-155, 150)
  point P141 (-155, 140)
  point P142 (-135, 380)
  point P143 (-155, 230)
  point P144 (-155, 240)
  point P145 (-155, 280)
  point P146 (-145, 230)
  point P147 (-135, 200)
  point P148 (-145, 140)
  point P149 (-155, 200)
  point P150 (-145, 200)
  point P151 (-155, 190)
  point P152 (-137, 412)
  point P153 (-137, 175.0655)
  point P154 (-190, 30)
  point P155 (-190, 90)
  point P156 (-190, 30)
  point P157 (-170, 90)
  point P158 (-190, 80)
  point P159 (-180, 90)
  point P160 (-180, 30)
  point P161 (-190, 40)
  point P162 (-172, 155.0655)
  point P163 (-172, 392)
  point P164 (-190, 120)
  point P165 (-190, 130)
  point P166 (-180, 120)
  point P167 (-190, 180)
  point P168 (-170, 180)
  point P169 (-190, 170)
  point P170 (-180, 180)
  point P171 (-190, 210)
  point P172 (-190, 220)
  point P173 (-180, 210)
  point P174 (-190, 270)
  point P175 (-170, 270)
  point P176 (-190, 260)
  point P177 (-180, 270)
  point P178 (-180, 300)
  point P179 (-190, 300)
  point P180 (-190, 310)
  point P181 (-170, 360)
  point P182 (-180, 360)
  point P183 (-190, 360)
  point P184 (-190, 350)
  point P185 (-180, 390)
  point P186 (-190, 390)
  point P187 (-190, 400)
  point P188 (-190, 440)
  point P189 (-190, 450)
  point P190 (-180, 450)
  point P191 (-170, 450)
  point P192 (-225, 50)
  point P193 (-225, 420)
  point P194 (-225, 470)
  point P195 (-205, 470)
  point P196 (-225, 460)
  point P197 (-215, 470)
  point P198 (-215, 50)
  point P199 (-225, 50)
  dimension "d0" = 20
  dimension "d1" = 60
  dimension "d2" = 10
  dimension "d3" = 10
  dimension "d4" = 10
  dimension "d5" = 10
  dimension "d6" = 2
  dimension "d22" = 20
  dimension "d23" = 60
  dimension "d24" = 10
  dimension "d25" = 10
  dimension "d26" = 10
  dimension "d27" = 10
  dimension "d28" = 2
  dimension "d29" = 20
  dimension "d30" = 60
  dimension "d31" = 10
  dimension "d32" = 10
  dimension "d33" = 10
  dimension "d34" = 10
  dimension "d35" = 2
  dimension "d36" = 20
  dimension "d37" = 60
  dimension "d38" = 10
  dimension "d39" = 10
  dimension "d40" = 10
  dimension "d41" = 10
  dimension "d42" = 2
  dimension "d43" = 20
  dimension "d44" = 60
  dimension "d45" = 10
  dimension "d46" = 10
  dimension "d47" = 10
  dimension "d48" = 10
  dimension "d49" = 2
  dimension "d464" = 500
  dimension "d465" = 52
  dimension "d466" = 30
  dimension "d467" = 30
  dimension "d468" = 50
  dimension "d469" = 20
  dimension "d470" = 60
  dimension "d471" = 10
  dimension "d472" = 10
  dimension "d473" = 10
  dimension "d474" = 10
  dimension "d475" = 2
  dimension "d476" = 20
  dimension "d477" = 60
  dimension "d478" = 10
  dimension "d479" = 10
  dimension "d480" = 10
  dimension "d481" = 10
  dimension "d482" = 2
  dimension "d483" = 20
  dimension "d484" = 60
  dimension "d485" = 10
  dimension "d486" = 10
  dimension "d487" = 10
  dimension "d488" = 10
  dimension "d489" = 2
  dimension "d490" = 20
  dimension "d491" = 60
  dimension "d492" = 10
  constraints: 560 point on line, 488 end point, 480 point on circle, 480 tangent, 240 centre point, 200 equal radius, 82 parallel, 41 horizontal, 41 perpendicular
  measures "d0" distance of point (-50, 90) point (-30, 90)
  measures "d1" distance of point (-50, 30) point (-50, 90)
  measures "d2" distance of point (-50, 80) point (-50, 90)
  measures "d3" distance of point (-40, 90) point (-50, 90)
  measures "d4" distance of point (-40, 30) point (-50, 30)
  measures "d5" distance of point (-50, 40) point (-50, 30)
  measures "d6" radius of A0
  measures "d22" distance of point (-50, 180) point (-30, 180)
  measures "d23" distance of point (-50, 120) point (-50, 180)
  measures "d24" distance of point (-50, 170) point (-50, 180)
  measures "d25" distance of point (-40, 180) point (-50, 180)
  measures "d26" distance of point (-40, 120) point (-50, 120)
  measures "d27" distance of point (-50, 130) point (-50, 120)
  measures "d28" radius of A6
  measures "d29" distance of point (-50, 270) point (-30, 270)
  measures "d30" distance of point (-50, 210) point (-50, 270)
  measures "d31" distance of point (-50, 260) point (-50, 270)
  measures "d32" distance of point (-40, 270) point (-50, 270)
  measures "d33" distance of point (-40, 210) point (-50, 210)
  measures "d34" distance of point (-50, 220) point (-50, 210)
  measures "d35" radius of A12
  measures "d36" distance of point (-50, 360) point (-30, 360)
  measures "d37" distance of point (-50, 300) point (-50, 360)
  measures "d38" distance of point (-50, 350) point (-50, 360)
  measures "d39" distance of point (-40, 360) point (-50, 360)
  measures "d40" distance of point (-40, 300) point (-50, 300)
  measures "d41" distance of point (-50, 310) point (-50, 300)
  measures "d42" radius of A23
  measures "d43" distance of point (-50, 450) point (-30, 450)
  measures "d44" distance of point (-50, 390) point (-50, 450)
  measures "d45" distance of point (-50, 440) point (-50, 450)
  measures "d46" distance of point (-40, 450) point (-50, 450)
  measures "d47" distance of point (-40, 390) point (-50, 390)
  measures "d48" distance of point (-50, 400) point (-50, 390)
  measures "d49" radius of A28
  measures "d464" distance of L30.end L31.end
  measures "d465" distance from line of A29.centre L32
  measures "d466" distance between parallel lines of L30 L0
  measures "d467" distance between parallel lines of L33 L21
  measures "d468" distance from line of L33 point (-50, 450)
  measures "d469" distance of point (-85, 110) point (-65, 110)
  measures "d470" distance of point (-85, 50) point (-85, 110)
  measures "d471" distance of point (-85, 100) point (-85, 110)
  measures "d472" distance of point (-75, 110) point (-85, 110)
  measures "d473" distance of point (-75, 50) point (-85, 50)
  measures "d474" distance of point (-85, 60) point (-85, 50)
  measures "d475" radius of A30
  measures "d476" distance of point (-85, 200) point (-65, 200)
  measures "d477" distance of point (-85, 140) point (-85, 200)
  measures "d478" distance of point (-85, 190) point (-85, 200)
  measures "d479" distance of point (-75, 200) point (-85, 200)
  measures "d480" distance of point (-75, 140) point (-85, 140)
  measures "d481" distance of point (-85, 150) point (-85, 140)
  measures "d482" radius of A41
  measures "d483" distance of point (-85, 290) point (-65, 290)
  measures "d484" distance of point (-85, 230) point (-85, 290)
  measures "d485" distance of point (-85, 280) point (-85, 290)
  measures "d486" distance of point (-75, 290) point (-85, 290)
  measures "d487" distance of point (-75, 230) point (-85, 230)
  measures "d488" distance of point (-85, 240) point (-85, 230)
  measures "d489" radius of A47
  measures "d490" distance of point (-85, 380) point (-65, 380)
  measures "d491" distance of point (-85, 320) point (-85, 380)
  measures "d492" distance of point (-85, 370) point (-85, 380)
extrude "Extrusion1" add sketch "Sketch1" along normal blind 10
equation "\"d3\" = d2"
equation "\"d4\" = d2"
equation "\"d5\" = d4"
equation "\"d25\" = d24"
equation "\"d26\" = d24"
equation "\"d27\" = d26"
equation "\"d32\" = d31"
equation "\"d33\" = d31"
equation "\"d34\" = d33"
equation "\"d39\" = d38"
equation "\"d40\" = d38"
equation "\"d41\" = d40"
equation "\"d46\" = d45"
equation "\"d47\" = d45"
equation "\"d48\" = d47"
equation "\"d472\" = d471"
equation "\"d473\" = d471"
equation "\"d474\" = d473"
equation "\"d479\" = d478"
equation "\"d480\" = d478"
equation "\"d481\" = d480"
equation "\"d486\" = d485"
equation "\"d487\" = d485"
equation "\"d488\" = d487"
body "Solid1"
